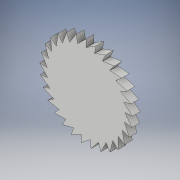
# Autodesk Inventor part: Ratchet Gear
Saved by Autodesk Inventor 2019 (Build 230136000, 136)
## iProperties
Created: 2020-05-30
Part Number: Ratchet Gear
Material: Generic
Document SubType Name: Modeling
Designer: 18186
Density: 1 g/cm^3
Appearance: Default
Author: 18186
Autodesk Inventor part; units mm, degrees
ref_plane "YZ Plane" through (0, 0, 0) normal (1, 0, 0) x (0, 1, 0)
ref_plane "XZ Plane" through (0, 0, 0) normal (0, 1, 0) x (-1, 0, 0)
ref_plane "XY Plane" through (0, 0, 0) normal (0, 0, 1) x (1, 0, 0)
sketch "Sketch1" plane through (0, 0, 0) normal (0, 0, 1) x (1, 0, 0)
  line L0 (0.009, 12.7) -> (0.009, 15.0802)
  line L1 (0.009, 15.0802) -> (3.5843, 15.0802) construction
  line L2 (0.009, 15.0802) -> (-2.651, 12.4202)
  line L3 (0.009, 15.0802) -> (3.7708, 15.0802) construction
  line L4 (-3.233, 14.7296) -> (-5.259, 11.56)
  line L5 (-2.7213, 12.405) -> (-3.233, 14.7296)
  line L6 (-6.3238, 13.6902) -> (-7.6211, 10.1592)
  line L7 (-5.3244, 11.53) -> (-6.3238, 13.6902)
  line L8 (-9.119, 12.0107) -> (-9.6268, 8.2834)
  line L9 (-7.6785, 10.1158) -> (-9.119, 12.0107)
  line L10 (-11.4877, 9.7696) -> (-11.1824, 6.0202)
  line L11 (-9.6736, 8.2287) -> (-11.4877, 9.7696)
  line L12 (-13.3193, 7.0716) -> (-12.2152, 3.4756)
  line L13 (-11.2164, 5.9567) -> (-13.3193, 7.0716)
  line L14 (-14.5281, 4.0431) -> (-12.6767, 0.7684)
  line L15 (-12.2347, 3.4063) -> (-14.5281, 4.0431)
  line L16 (-15.0576, 0.8254) -> (-12.5455, -1.9747)
  line L17 (-12.6809, 0.6966) -> (-15.0576, 0.8254)
  line L18 (-14.883, -2.4308) -> (-11.8277, -4.6254)
  line L19 (-12.5342, -2.0457) -> (-14.883, -2.4308)
  line L20 (-14.0125, -5.5734) -> (-10.5569, -7.0599)
  line L21 (-11.8013, -4.6924) -> (-14.0125, -5.5734)
  line L22 (-12.4868, -8.4554) -> (-8.7924, -9.1643)
  line L23 (-10.5167, -7.1196) -> (-12.4868, -8.4554)
  line L24 (-10.3772, -10.942) -> (-6.6168, -10.8401)
  line L25 (-8.7403, -9.2139) -> (-10.3772, -10.942)
  line L26 (-7.7824, -12.9169) -> (-4.1318, -12.0091)
  line L27 (-6.5552, -10.8774) -> (-7.7824, -12.9169)
  line L28 (-4.8237, -14.2879) -> (-1.4536, -12.6165)
  line L29 (-4.0637, -12.0323) -> (-4.8237, -14.2879)
  line L30 (-1.6394, -14.9908) -> (1.2926, -12.6341)
  line L31 (-1.3821, -12.6246) -> (-1.6394, -14.9908)
  line L32 (1.6215, -14.9928) -> (3.9783, -12.0608)
  line L33 (1.3642, -12.6265) -> (1.6215, -14.9928)
  line L34 (4.8066, -14.2937) -> (6.478, -10.9236)
  line L35 (4.0466, -12.0381) -> (4.8066, -14.2937)
  line L36 (7.7669, -12.9262) -> (8.6748, -9.2757)
  line L37 (6.5398, -10.8867) -> (7.7669, -12.9262)
  line L38 (10.3641, -10.9544) -> (10.466, -7.194)
  line L39 (8.7272, -9.2263) -> (10.3641, -10.9544)
  line L40 (12.4767, -8.4703) -> (11.7678, -4.7759)
  line L41 (10.5066, -7.1345) -> (12.4767, -8.4703)
  line L42 (14.0058, -5.5901) -> (12.5193, -2.1345)
  line L43 (11.7947, -4.7091) -> (14.0058, -5.5901)
  line L44 (14.8801, -2.4486) -> (12.6855, 0.6067)
  line L45 (12.5312, -2.0635) -> (14.8801, -2.4486)
  line L46 (15.0586, 0.8074) -> (12.2585, 3.3195)
  line L47 (12.6819, 0.6786) -> (15.0586, 0.8074)
  line L48 (14.5329, 4.0257) -> (11.2583, 5.8771)
  line L49 (12.2395, 3.3889) -> (14.5329, 4.0257)
  line L50 (13.3278, 7.0557) -> (9.7317, 8.1599)
  line L51 (11.2248, 5.9408) -> (13.3278, 7.0557)
  line L52 (11.4994, 9.7559) -> (7.75, 10.0612)
  line L53 (9.6853, 8.2149) -> (11.4994, 9.7559)
  line L54 (9.1333, 11.9998) -> (5.406, 11.492)
  line L55 (7.6929, 10.1049) -> (9.1333, 11.9998)
  line L56 (6.3402, 13.6826) -> (2.8092, 12.3854)
  line L57 (5.3408, 11.5224) -> (6.3402, 13.6826)
  line L58 (3.2506, 14.7257) -> (0.081, 12.6997)
  line L59 (2.7389, 12.4011) -> (3.2506, 14.7257)
  arc A0 (-2.651, 12.4202) -> (-2.7213, 12.405) centre (0, 0) ccw
  arc A1 (0.081, 12.6997) -> (0.009, 12.7) centre (0, 0) ccw
  arc A2 (2.8092, 12.3854) -> (2.7389, 12.4011) centre (0, 0) ccw
  arc A3 (5.406, 11.492) -> (5.3408, 11.5224) centre (0, 0) ccw
  arc A4 (7.75, 10.0612) -> (7.6929, 10.1049) centre (0, 0) ccw
  arc A5 (9.7317, 8.1599) -> (9.6853, 8.2149) centre (0, 0) ccw
  arc A6 (11.2583, 5.8771) -> (11.2248, 5.9408) centre (0, 0) ccw
  arc A7 (12.2585, 3.3195) -> (12.2395, 3.3889) centre (0, 0) ccw
  arc A8 (12.6855, 0.6067) -> (12.6819, 0.6786) centre (0, 0) ccw
  arc A9 (12.5193, -2.1345) -> (12.5312, -2.0635) centre (0, 0) ccw
  arc A10 (11.7678, -4.7759) -> (11.7947, -4.7091) centre (0, 0) ccw
  arc A11 (10.466, -7.194) -> (10.5066, -7.1345) centre (0, 0) ccw
  arc A12 (8.6748, -9.2757) -> (8.7272, -9.2263) centre (0, 0) ccw
  arc A13 (6.478, -10.9236) -> (6.5398, -10.8867) centre (0, 0) ccw
  arc A14 (3.9783, -12.0608) -> (4.0466, -12.0381) centre (0, 0) ccw
  arc A15 (1.2926, -12.6341) -> (1.3642, -12.6265) centre (0, 0) ccw
  arc A16 (-1.4536, -12.6165) -> (-1.3821, -12.6246) centre (0, 0) ccw
  arc A17 (-4.1318, -12.0091) -> (-4.0637, -12.0323) centre (0, 0) ccw
  arc A18 (-6.6168, -10.8401) -> (-6.5552, -10.8774) centre (0, 0) ccw
  arc A19 (-8.7924, -9.1643) -> (-8.7403, -9.2139) centre (0, 0) ccw
  arc A20 (-10.5569, -7.0599) -> (-10.5167, -7.1196) centre (0, 0) ccw
  arc A21 (-11.8277, -4.6254) -> (-11.8013, -4.6924) centre (0, 0) ccw
  arc A22 (-12.5455, -1.9747) -> (-12.5342, -2.0457) centre (0, 0) ccw
  arc A23 (-12.6767, 0.7684) -> (-12.6809, 0.6966) centre (0, 0) ccw
  arc A24 (-12.2152, 3.4756) -> (-12.2347, 3.4063) centre (0, 0) ccw
  arc A25 (-11.1824, 6.0202) -> (-11.2164, 5.9567) centre (0, 0) ccw
  arc A26 (-9.6268, 8.2834) -> (-9.6736, 8.2287) centre (0, 0) ccw
  arc A27 (-5.259, 11.56) -> (-5.3244, 11.53) centre (0, 0) ccw
  arc A28 (-7.6211, 10.1592) -> (-7.6785, 10.1158) centre (0, 0) ccw
  dimension "d2" = 135
  dimension "d5" = 360
  constraints: 120 end point, 2 horizontal, 1 equal length, 1 vertical, 234 other
  measures "d2" angle of L2 L3
extrude "Extrusion1" add sketch "Sketch1" along normal blind 2.54
body "Solid1"
